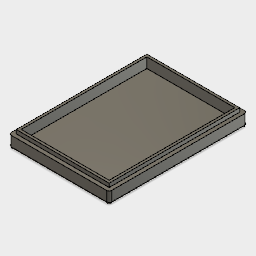
LED_top (Autodesk Fusion 360 design; units mm, degrees)
Autodesk Fusion 360 part; units mm, degrees
sketch "Sketch1" plane through (0, 0, 0) normal (0, 1, 0) x (1, 0, 0)
  line L0 (0, 0) -> (80, 0)
  line L1 (80, 0) -> (80, 110)
  line L2 (80, 110) -> (0, 110)
  line L3 (0, 110) -> (0, 0)
extrude "Extrude1" add sketch "Sketch1" along normal blind 10
shell "Shell1" thickness 5 removed faces 1 at (26.6667, 10, -73.3333)
fillet "Fillet3" radius 2 5 edges at (80, 5, -110) (40, 0, -110) (0, 5, -110) (0, 0, -55) (0, 5, 0)
fillet "Fillet4" radius 2 5 edges at (0.5858, 0.5858, -0.5858) (41, 0, 0) (80, 5, 0) (80, 0, -54) (79.4142, 0.5858, -109.4142)
sketch "Sketch4" plane through (0, 10, 0) normal (0, 1, 0) x (-1, 0, 0)
  line L0 (-5, -105) -> (-75, -105)
  line L1 (-75, -105) -> (-75, -5)
  line L2 (-75, -5) -> (-5, -5)
  line L3 (-5, -5) -> (-5, -105)
  arc A0 (-78, 0) -> (-80, -2) centre (-78, -2) ccw
  line L4 (-80, -2) -> (-80, -108)
  arc A1 (-80, -108) -> (-78, -110) centre (-78, -108) ccw
  line L5 (-78, -110) -> (-2, -110)
  arc A2 (-2, -110) -> (0, -108) centre (-2, -108) ccw
  line L6 (0, -108) -> (0, -2)
  arc A3 (0, -2) -> (-2, 0) centre (-2, -2) ccw
  line L7 (-2, 0) -> (-78, 0)
  line L8 (-3, -3) -> (-77, -3)
  line L9 (-77, -3) -> (-77, -107)
  line L10 (-77, -107) -> (-3, -107)
  line L11 (-3, -107) -> (-3, -3)
extrude "Extrude3" add sketch "Sketch4" along normal blind 3 contours L8 L9 L10 L11
